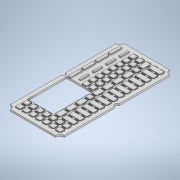
# Autodesk Inventor part: Backboard
Saved by Autodesk Inventor 2021 (Build 250183000, 183)
## iProperties
Created: 2020-06-05
Part Number: Backboard
Material: Generic
Document SubType Name: Modeling
Designer: ameli
Density: 1 g/cm^3
Appearance: Default
Author: ameli
Autodesk Inventor part; units mm, degrees
(part 1 of 3)
ref_plane "YZ Plane" through (0, 0, 0) normal (1, 0, 0) x (0, 1, 0)
ref_plane "XZ Plane" through (0, 0, 0) normal (0, 1, 0) x (-1, 0, 0)
ref_plane "XY Plane" through (0, 0, 0) normal (0, 0, 1) x (1, 0, 0)
sketch "Sketch1" plane through (0, 0, 0) normal (0, 1, 0) x (-1, 0, 0)
  line L0 (60.5, 128.5) -> (-60.5, 128.5)
  line L1 (-60.5, 128.5) -> (-60.5, -128.5)
  line L2 (-60.5, -128.5) -> (60.5, -128.5)
  line L3 (60.5, -128.5) -> (60.5, 128.5)
  point P0 (0, 0)
  dimension "d0" = 121
  dimension "d1" = 257
  dimension "d2" = 60.5
  dimension "d3" = 128.5
  constraints: 8 end point, 2 parallel, 1 horizontal, 1 perpendicular
  measures "d0" distance of L0.start L0.end
  measures "d1" distance of L2.end L0.start
  measures "d2" distance from line of point (0, 0) L3
  measures "d3" distance from line of point (0, 0) L0
extrude "Extrusion1" add sketch "Sketch1" along normal blind 4
sketch "Sketch6" plane through (0, 4, 0) normal (0, 1, 0) x (1, 0, 0)
  line L0 (-52, -89.5) -> (7, -89.5)
  line L1 (7, -89.5) -> (7, -0.5)
  line L2 (7, -0.5) -> (-52, -0.5)
  line L3 (-52, -0.5) -> (-52, -89.5)
  line L4 (-60.5, 128.5) -> (-60.5, -128.5) projected
  line L5 (-60.5, -128.5) -> (60.5, -128.5) projected
  point P0 (0, 0)
  dimension "d22" = 89
  dimension "d23" = 59
  dimension "d24" = 8.5
  dimension "d336" = 39
  constraints: 8 end point, 2 parallel, 1 horizontal, 1 perpendicular
  measures "d22" distance of L2.end L0.start
  measures "d23" distance of L0.start L0.end
  measures "d24" distance between parallel lines of L4 L3
  measures "d336" distance between parallel lines of L5 L0
extrude "Extrusion2" cut sketch "Sketch6" against normal blind 10
sketch "Sketch10" plane through (0, 4, 0) normal (0, 1, 0) x (1, 0, 0)
  line L0 (-49.25, -119.5) -> (-40.75, -119.5)
  line L1 (-40.75, -119.5) -> (-40.75, -118)
  line L2 (-40.75, -118) -> (-49.25, -118)
  line L3 (-49.25, -118) -> (-49.25, -119.5)
  line L4 (-49.25, -107) -> (-40.75, -107)
  line L5 (-40.75, -107) -> (-40.75, -105.5)
  line L6 (-40.75, -105.5) -> (-49.25, -105.5)
  line L7 (-49.25, -105.5) -> (-49.25, -107)
  line L8 (-60.5, 128.5) -> (-60.5, -128.5) projected
  line L9 (-60.5, -128.5) -> (60.5, -128.5) projected
  line L10 (-49.25, -104.5) -> (-40.75, -104.5)
  line L11 (-40.75, -104.5) -> (-40.75, -103)
  line L12 (-40.75, -103) -> (-49.25, -103)
  line L13 (-49.25, -103) -> (-49.25, -104.5)
  line L14 (-49.25, -92) -> (-40.75, -92)
  line L15 (-40.75, -92) -> (-40.75, -90.5)
  line L16 (-40.75, -90.5) -> (-49.25, -90.5)
  line L17 (-49.25, -90.5) -> (-49.25, -92)
  line L18 (-49.25, -89.5) -> (-40.75, -89.5)
  line L19 (-40.75, -89.5) -> (-40.75, -88)
  line L20 (-40.75, -88) -> (-49.25, -88)
  line L21 (-49.25, -88) -> (-49.25, -89.5)
  line L22 (-49.25, -77) -> (-40.75, -77)
  line L23 (-40.75, -77) -> (-40.75, -75.5)
  line L24 (-40.75, -75.5) -> (-49.25, -75.5)
  line L25 (-49.25, -75.5) -> (-49.25, -77)
  line L26 (-49.25, -74.5) -> (-40.75, -74.5)
  line L27 (-40.75, -74.5) -> (-40.75, -73)
  line L28 (-40.75, -73) -> (-49.25, -73)
  line L29 (-49.25, -73) -> (-49.25, -74.5)
  line L30 (-49.25, -62) -> (-40.75, -62)
  line L31 (-40.75, -62) -> (-40.75, -60.5)
  line L32 (-40.75, -60.5) -> (-49.25, -60.5)
  line L33 (-49.25, -60.5) -> (-49.25, -62)
  line L34 (-49.25, -59.5) -> (-40.75, -59.5)
  line L35 (-40.75, -59.5) -> (-40.75, -58)
  line L36 (-40.75, -58) -> (-49.25, -58)
  line L37 (-49.25, -58) -> (-49.25, -59.5)
  line L38 (-49.25, -47) -> (-40.75, -47)
  line L39 (-40.75, -47) -> (-40.75, -45.5)
  line L40 (-40.75, -45.5) -> (-49.25, -45.5)
  line L41 (-49.25, -45.5) -> (-49.25, -47)
  line L42 (-49.25, -44.5) -> (-40.75, -44.5)
  line L43 (-40.75, -44.5) -> (-40.75, -43)
  line L44 (-40.75, -43) -> (-49.25, -43)
  line L45 (-49.25, -43) -> (-49.25, -44.5)
  line L46 (-49.25, -32) -> (-40.75, -32)
  line L47 (-40.75, -32) -> (-40.75, -30.5)
  line L48 (-40.75, -30.5) -> (-49.25, -30.5)
  line L49 (-49.25, -30.5) -> (-49.25, -32)
  line L50 (-49.25, -29.5) -> (-40.75, -29.5)
  line L51 (-40.75, -29.5) -> (-40.75, -28)
  line L52 (-40.75, -28) -> (-49.25, -28)
  line L53 (-49.25, -28) -> (-49.25, -29.5)
  line L54 (-49.25, -17) -> (-40.75, -17)
  line L55 (-40.75, -17) -> (-40.75, -15.5)
  line L56 (-40.75, -15.5) -> (-49.25, -15.5)
  line L57 (-49.25, -15.5) -> (-49.25, -17)
  line L58 (-49.25, -14.5) -> (-40.75, -14.5)
  line L59 (-40.75, -14.5) -> (-40.75, -13)
  line L60 (-40.75, -13) -> (-49.25, -13)
  line L61 (-49.25, -13) -> (-49.25, -14.5)
  line L62 (-49.25, -2) -> (-40.75, -2)
  line L63 (-40.75, -2) -> (-40.75, -0.5)
  line L64 (-40.75, -0.5) -> (-49.25, -0.5)
  line L65 (-49.25, -0.5) -> (-49.25, -2)
  line L66 (-49.25, 0.5) -> (-40.75, 0.5)
  line L67 (-40.75, 0.5) -> (-40.75, 2)
  line L68 (-40.75, 2) -> (-49.25, 2)
  line L69 (-49.25, 2) -> (-49.25, 0.5)
  line L70 (-49.25, 13) -> (-40.75, 13)
  line L71 (-40.75, 13) -> (-40.75, 14.5)
  line L72 (-40.75, 14.5) -> (-49.25, 14.5)
  line L73 (-49.25, 14.5) -> (-49.25, 13)
  line L74 (-49.25, 15.5) -> (-40.75, 15.5)
  line L75 (-40.75, 15.5) -> (-40.75, 17)
  line L76 (-40.75, 17) -> (-49.25, 17)
  line L77 (-49.25, 17) -> (-49.25, 15.5)
  line L78 (-49.25, 28) -> (-40.75, 28)
  line L79 (-40.75, 28) -> (-40.75, 29.5)
  line L80 (-40.75, 29.5) -> (-49.25, 29.5)
  line L81 (-49.25, 29.5) -> (-49.25, 28)
  line L82 (-49.25, 30.5) -> (-40.75, 30.5)
  line L83 (-40.75, 30.5) -> (-40.75, 32)
  line L84 (-40.75, 32) -> (-49.25, 32)
  line L85 (-49.25, 32) -> (-49.25, 30.5)
  line L86 (-49.25, 43) -> (-40.75, 43)
  line L87 (-40.75, 43) -> (-40.75, 44.5)
  line L88 (-40.75, 44.5) -> (-49.25, 44.5)
  line L89 (-49.25, 44.5) -> (-49.25, 43)
  line L90 (-49.25, 45.5) -> (-40.75, 45.5)
  line L91 (-40.75, 45.5) -> (-40.75, 47)
  line L92 (-40.75, 47) -> (-49.25, 47)
  line L93 (-49.25, 47) -> (-49.25, 45.5)
  line L94 (-49.25, 58) -> (-40.75, 58)
  line L95 (-40.75, 58) -> (-40.75, 59.5)
  line L96 (-40.75, 59.5) -> (-49.25, 59.5)
  line L97 (-49.25, 59.5) -> (-49.25, 58)
  line L98 (-49.25, 60.5) -> (-40.75, 60.5)
  line L99 (-40.75, 60.5) -> (-40.75, 62)
  line L100 (-40.75, 62) -> (-49.25, 62)
  line L101 (-49.25, 62) -> (-49.25, 60.5)
  line L102 (-49.25, 73) -> (-40.75, 73)
  line L103 (-40.75, 73) -> (-40.75, 74.5)
  line L104 (-40.75, 74.5) -> (-49.25, 74.5)
  line L105 (-49.25, 74.5) -> (-49.25, 73)
  line L106 (-49.25, 75.5) -> (-40.75, 75.5)
  line L107 (-40.75, 75.5) -> (-40.75, 77)
  line L108 (-40.75, 77) -> (-49.25, 77)
  line L109 (-49.25, 77) -> (-49.25, 75.5)
  line L110 (-49.25, 88) -> (-40.75, 88)
  line L111 (-40.75, 88) -> (-40.75, 89.5)
  line L112 (-40.75, 89.5) -> (-49.25, 89.5)
  line L113 (-49.25, 89.5) -> (-49.25, 88)
  line L114 (-49.25, 90.5) -> (-40.75, 90.5)
  line L115 (-40.75, 90.5) -> (-40.75, 92)
  line L116 (-40.75, 92) -> (-49.25, 92)
  line L117 (-49.25, 92) -> (-49.25, 90.5)
  line L118 (-49.25, 103) -> (-40.75, 103)
  line L119 (-40.75, 103) -> (-40.75, 104.5)
  line L120 (-40.75, 104.5) -> (-49.25, 104.5)
  line L121 (-49.25, 104.5) -> (-49.25, 103)
  line L122 (-49.25, 105.5) -> (-40.75, 105.5)
  line L123 (-40.75, 105.5) -> (-40.75, 107)
  line L124 (-40.75, 107) -> (-49.25, 107)
  line L125 (-49.25, 107) -> (-49.25, 105.5)
  line L126 (-49.25, 118) -> (-40.75, 118)
  line L127 (-40.75, 118) -> (-40.75, 119.5)
  line L128 (-40.75, 119.5) -> (-49.25, 119.5)
  line L129 (-49.25, 119.5) -> (-49.25, 118)
  line L130 (-34.25, -119.5) -> (-25.75, -119.5)
  line L131 (-25.75, -119.5) -> (-25.75, -118)
  line L132 (-25.75, -118) -> (-34.25, -118)
  line L133 (-34.25, -118) -> (-34.25, -119.5)
  line L134 (-34.25, -107) -> (-25.75, -107)
  line L135 (-25.75, -107) -> (-25.75, -105.5)
  line L136 (-25.75, -105.5) -> (-34.25, -105.5)
  line L137 (-34.25, -105.5) -> (-34.25, -107)
  line L138 (-34.25, -104.5) -> (-25.75, -104.5)
  line L139 (-25.75, -104.5) -> (-25.75, -103)
  line L140 (-25.75, -103) -> (-34.25, -103)
  line L141 (-34.25, -103) -> (-34.25, -104.5)
  line L142 (-34.25, -92) -> (-25.75, -92)
  line L143 (-25.75, -92) -> (-25.75, -90.5)
  line L144 (-25.75, -90.5) -> (-34.25, -90.5)
  line L145 (-34.25, -90.5) -> (-34.25, -92)
  line L146 (-34.25, -89.5) -> (-25.75, -89.5)
  line L147 (-25.75, -89.5) -> (-25.75, -88)
  line L148 (-25.75, -88) -> (-34.25, -88)
  line L149 (-34.25, -88) -> (-34.25, -89.5)
  line L150 (-34.25, -77) -> (-25.75, -77)
  line L151 (-25.75, -77) -> (-25.75, -75.5)
  line L152 (-25.75, -75.5) -> (-34.25, -75.5)
  line L153 (-34.25, -75.5) -> (-34.25, -77)
  line L154 (-34.25, -74.5) -> (-25.75, -74.5)
  line L155 (-25.75, -74.5) -> (-25.75, -73)
  line L156 (-25.75, -73) -> (-34.25, -73)
  line L157 (-34.25, -73) -> (-34.25, -74.5)
  line L158 (-34.25, -62) -> (-25.75, -62)
  line L159 (-25.75, -62) -> (-25.75, -60.5)
  line L160 (-25.75, -60.5) -> (-34.25, -60.5)
  line L161 (-34.25, -60.5) -> (-34.25, -62)
  line L162 (-34.25, -59.5) -> (-25.75, -59.5)
  line L163 (-25.75, -59.5) -> (-25.75, -58)
  line L164 (-25.75, -58) -> (-34.25, -58)
  line L165 (-34.25, -58) -> (-34.25, -59.5)
  line L166 (-34.25, -47) -> (-25.75, -47)
  line L167 (-25.75, -47) -> (-25.75, -45.5)
  line L168 (-25.75, -45.5) -> (-34.25, -45.5)
  line L169 (-34.25, -45.5) -> (-34.25, -47)
  line L170 (-34.25, -44.5) -> (-25.75, -44.5)
  line L171 (-25.75, -44.5) -> (-25.75, -43)
  line L172 (-25.75, -43) -> (-34.25, -43)
  line L173 (-34.25, -43) -> (-34.25, -44.5)
  line L174 (-34.25, -32) -> (-25.75, -32)
  line L175 (-25.75, -32) -> (-25.75, -30.5)
  line L176 (-25.75, -30.5) -> (-34.25, -30.5)
  line L177 (-34.25, -30.5) -> (-34.25, -32)
  line L178 (-34.25, -29.5) -> (-25.75, -29.5)
  line L179 (-25.75, -29.5) -> (-25.75, -28)
  line L180 (-25.75, -28) -> (-34.25, -28)
  line L181 (-34.25, -28) -> (-34.25, -29.5)
  line L182 (-34.25, -17) -> (-25.75, -17)
  line L183 (-25.75, -17) -> (-25.75, -15.5)
  line L184 (-25.75, -15.5) -> (-34.25, -15.5)
  line L185 (-34.25, -15.5) -> (-34.25, -17)
  line L186 (-34.25, -14.5) -> (-25.75, -14.5)
  line L187 (-25.75, -14.5) -> (-25.75, -13)
  line L188 (-25.75, -13) -> (-34.25, -13)
  line L189 (-34.25, -13) -> (-34.25, -14.5)
  line L190 (-34.25, -2) -> (-25.75, -2)
  line L191 (-25.75, -2) -> (-25.75, -0.5)
  line L192 (-25.75, -0.5) -> (-34.25, -0.5)
  line L193 (-34.25, -0.5) -> (-34.25, -2)
  line L194 (-34.25, 0.5) -> (-25.75, 0.5)
  line L195 (-25.75, 0.5) -> (-25.75, 2)
  line L196 (-25.75, 2) -> (-34.25, 2)
  line L197 (-34.25, 2) -> (-34.25, 0.5)
  line L198 (-34.25, 13) -> (-25.75, 13)
  line L199 (-25.75, 13) -> (-25.75, 14.5)
  line L200 (-25.75, 14.5) -> (-34.25, 14.5)
  line L201 (-34.25, 14.5) -> (-34.25, 13)
  line L202 (-34.25, 15.5) -> (-25.75, 15.5)
  line L203 (-25.75, 15.5) -> (-25.75, 17)
  line L204 (-25.75, 17) -> (-34.25, 17)
  line L205 (-34.25, 17) -> (-34.25, 15.5)
  line L206 (-34.25, 28) -> (-25.75, 28)
  line L207 (-25.75, 28) -> (-25.75, 29.5)
  line L208 (-25.75, 29.5) -> (-34.25, 29.5)
  line L209 (-34.25, 29.5) -> (-34.25, 28)
  line L210 (-34.25, 30.5) -> (-25.75, 30.5)
  line L211 (-25.75, 30.5) -> (-25.75, 32)
  line L212 (-25.75, 32) -> (-34.25, 32)
  line L213 (-34.25, 32) -> (-34.25, 30.5)
  line L214 (-34.25, 43) -> (-25.75, 43)
  line L215 (-25.75, 43) -> (-25.75, 44.5)
  line L216 (-25.75, 44.5) -> (-34.25, 44.5)
  line L217 (-34.25, 44.5) -> (-34.25, 43)
  line L218 (-34.25, 45.5) -> (-25.75, 45.5)
  line L219 (-25.75, 45.5) -> (-25.75, 47)
  line L220 (-25.75, 47) -> (-34.25, 47)
  line L221 (-34.25, 47) -> (-34.25, 45.5)
  line L222 (-34.25, 58) -> (-25.75, 58)
  line L223 (-25.75, 58) -> (-25.75, 59.5)
  line L224 (-25.75, 59.5) -> (-34.25, 59.5)
  line L225 (-34.25, 59.5) -> (-34.25, 58)
  line L226 (-34.25, 60.5) -> (-25.75, 60.5)
  line L227 (-25.75, 60.5) -> (-25.75, 62)
  line L228 (-25.75, 62) -> (-34.25, 62)
  line L229 (-34.25, 62) -> (-34.25, 60.5)
  line L230 (-34.25, 73) -> (-25.75, 73)
  line L231 (-25.75, 73) -> (-25.75, 74.5)
  line L232 (-25.75, 74.5) -> (-34.25, 74.5)
  line L233 (-34.25, 74.5) -> (-34.25, 73)
  line L234 (-34.25, 75.5) -> (-25.75, 75.5)
  line L235 (-25.75, 75.5) -> (-25.75, 77)
  line L236 (-25.75, 77) -> (-34.25, 77)
  line L237 (-34.25, 77) -> (-34.25, 75.5)
  line L238 (-34.25, 88) -> (-25.75, 88)
  line L239 (-25.75, 88) -> (-25.75, 89.5)
  line L240 (-25.75, 89.5) -> (-34.25, 89.5)
  line L241 (-34.25, 89.5) -> (-34.25, 88)
  line L242 (-34.25, 90.5) -> (-25.75, 90.5)
  line L243 (-25.75, 90.5) -> (-25.75, 92)
  line L244 (-25.75, 92) -> (-34.25, 92)
  line L245 (-34.25, 92) -> (-34.25, 90.5)
  line L246 (-34.25, 103) -> (-25.75, 103)
  line L247 (-25.75, 103) -> (-25.75, 104.5)
  line L248 (-25.75, 104.5) -> (-34.25, 104.5)
  line L249 (-34.25, 104.5) -> (-34.25, 103)
  line L250 (-34.25, 105.5) -> (-25.75, 105.5)
  line L251 (-25.75, 105.5) -> (-25.75, 107)
  line L252 (-25.75, 107) -> (-34.25, 107)
  line L253 (-34.25, 107) -> (-34.25, 105.5)
  line L254 (-34.25, 118) -> (-25.75, 118)
  line L255 (-25.75, 118) -> (-25.75, 119.5)
  line L256 (-25.75, 119.5) -> (-34.25, 119.5)
  line L257 (-34.25, 119.5) -> (-34.25, 118)
  line L258 (-19.25, -119.5) -> (-10.75, -119.5)
  line L259 (-10.75, -119.5) -> (-10.75, -118)
  line L260 (-10.75, -118) -> (-19.25, -118)
  line L261 (-19.25, -118) -> (-19.25, -119.5)
  line L262 (-19.25, -107) -> (-10.75, -107)
  line L263 (-10.75, -107) -> (-10.75, -105.5)
  line L264 (-10.75, -105.5) -> (-19.25, -105.5)
  line L265 (-19.25, -105.5) -> (-19.25, -107)
  line L266 (-19.25, -104.5) -> (-10.75, -104.5)
  line L267 (-10.75, -104.5) -> (-10.75, -103)
  line L268 (-10.75, -103) -> (-19.25, -103)
  line L269 (-19.25, -103) -> (-19.25, -104.5)
  line L270 (-19.25, -92) -> (-10.75, -92)
  line L271 (-10.75, -92) -> (-10.75, -90.5)
  line L272 (-10.75, -90.5) -> (-19.25, -90.5)
  line L273 (-19.25, -90.5) -> (-19.25, -92)
  line L274 (-19.25, -89.5) -> (-10.75, -89.5)
  line L275 (-10.75, -89.5) -> (-10.75, -88)
  line L276 (-10.75, -88) -> (-19.25, -88)
  line L277 (-19.25, -88) -> (-19.25, -89.5)
  line L278 (-19.25, -77) -> (-10.75, -77)
  line L279 (-10.75, -77) -> (-10.75, -75.5)
  line L280 (-10.75, -75.5) -> (-19.25, -75.5)
  line L281 (-19.25, -75.5) -> (-19.25, -77)
  line L282 (-19.25, -74.5) -> (-10.75, -74.5)
  line L283 (-10.75, -74.5) -> (-10.75, -73)
  line L284 (-10.75, -73) -> (-19.25, -73)
  line L285 (-19.25, -73) -> (-19.25, -74.5)
  line L286 (-19.25, -62) -> (-10.75, -62)
  line L287 (-10.75, -62) -> (-10.75, -60.5)
  line L288 (-10.75, -60.5) -> (-19.25, -60.5)
  line L289 (-19.25, -60.5) -> (-19.25, -62)
  line L290 (-19.25, -59.5) -> (-10.75, -59.5)
  line L291 (-10.75, -59.5) -> (-10.75, -58)
  line L292 (-10.75, -58) -> (-19.25, -58)
  line L293 (-19.25, -58) -> (-19.25, -59.5)
  line L294 (-19.25, -47) -> (-10.75, -47)
  line L295 (-10.75, -47) -> (-10.75, -45.5)
  line L296 (-10.75, -45.5) -> (-19.25, -45.5)
  line L297 (-19.25, -45.5) -> (-19.25, -47)
  line L298 (-19.25, -44.5) -> (-10.75, -44.5)
  line L299 (-10.75, -44.5) -> (-10.75, -43)
  line L300 (-10.75, -43) -> (-19.25, -43)
  line L301 (-19.25, -43) -> (-19.25, -44.5)
  line L302 (-19.25, -32) -> (-10.75, -32)
  line L303 (-10.75, -32) -> (-10.75, -30.5)
  line L304 (-10.75, -30.5) -> (-19.25, -30.5)
  line L305 (-19.25, -30.5) -> (-19.25, -32)
  line L306 (-19.25, -29.5) -> (-10.75, -29.5)
  line L307 (-10.75, -29.5) -> (-10.75, -28)
  line L308 (-10.75, -28) -> (-19.25, -28)
  line L309 (-19.25, -28) -> (-19.25, -29.5)
  line L310 (-19.25, -17) -> (-10.75, -17)
  line L311 (-10.75, -17) -> (-10.75, -15.5)
  line L312 (-10.75, -15.5) -> (-19.25, -15.5)
  line L313 (-19.25, -15.5) -> (-19.25, -17)
  line L314 (-19.25, -14.5) -> (-10.75, -14.5)
  line L315 (-10.75, -14.5) -> (-10.75, -13)
  line L316 (-10.75, -13) -> (-19.25, -13)
  line L317 (-19.25, -13) -> (-19.25, -14.5)
  line L318 (-19.25, -2) -> (-10.75, -2)
  line L319 (-10.75, -2) -> (-10.75, -0.5)
  line L320 (-10.75, -0.5) -> (-19.25, -0.5)
  line L321 (-19.25, -0.5) -> (-19.25, -2)
  line L322 (-19.25, 0.5) -> (-10.75, 0.5)
  line L323 (-10.75, 0.5) -> (-10.75, 2)
  line L324 (-10.75, 2) -> (-19.25, 2)
  line L325 (-19.25, 2) -> (-19.25, 0.5)
  line L326 (-19.25, 13) -> (-10.75, 13)
  line L327 (-10.75, 13) -> (-10.75, 14.5)
  line L328 (-10.75, 14.5) -> (-19.25, 14.5)
  line L329 (-19.25, 14.5) -> (-19.25, 13)
  line L330 (-19.25, 15.5) -> (-10.75, 15.5)
  line L331 (-10.75, 15.5) -> (-10.75, 17)
  line L332 (-10.75, 17) -> (-19.25, 17)
  line L333 (-19.25, 17) -> (-19.25, 15.5)
  line L334 (-19.25, 28) -> (-10.75, 28)
  line L335 (-10.75, 28) -> (-10.75, 29.5)
  line L336 (-10.75, 29.5) -> (-19.25, 29.5)
  line L337 (-19.25, 29.5) -> (-19.25, 28)
  line L338 (-19.25, 30.5) -> (-10.75, 30.5)
  line L339 (-10.75, 30.5) -> (-10.75, 32)
  line L340 (-10.75, 32) -> (-19.25, 32)
  line L341 (-19.25, 32) -> (-19.25, 30.5)
  line L342 (-19.25, 43) -> (-10.75, 43)
  line L343 (-10.75, 43) -> (-10.75, 44.5)
  line L344 (-10.75, 44.5) -> (-19.25, 44.5)
  line L345 (-19.25, 44.5) -> (-19.25, 43)
  line L346 (-19.25, 45.5) -> (-10.75, 45.5)
  line L347 (-10.75, 45.5) -> (-10.75, 47)
  line L348 (-10.75, 47) -> (-19.25, 47)
  line L349 (-19.25, 47) -> (-19.25, 45.5)
  line L350 (-19.25, 58) -> (-10.75, 58)
  line L351 (-10.75, 58) -> (-10.75, 59.5)
  line L352 (-10.75, 59.5) -> (-19.25, 59.5)
  line L353 (-19.25, 59.5) -> (-19.25, 58)
  line L354 (-19.25, 60.5) -> (-10.75, 60.5)
  line L355 (-10.75, 60.5) -> (-10.75, 62)
  line L356 (-10.75, 62) -> (-19.25, 62)
  line L357 (-19.25, 62) -> (-19.25, 60.5)
  line L358 (-19.25, 73) -> (-10.75, 73)
  line L359 (-10.75, 73) -> (-10.75, 74.5)
  line L360 (-10.75, 74.5) -> (-19.25, 74.5)
  line L361 (-19.25, 74.5) -> (-19.25, 73)
  line L362 (-19.25, 75.5) -> (-10.75, 75.5)
  line L363 (-10.75, 75.5) -> (-10.75, 77)
  line L364 (-10.75, 77) -> (-19.25, 77)
  line L365 (-19.25, 77) -> (-19.25, 75.5)
  line L366 (-19.25, 88) -> (-10.75, 88)
  line L367 (-10.75, 88) -> (-10.75, 89.5)
  line L368 (-10.75, 89.5) -> (-19.25, 89.5)
  line L369 (-19.25, 89.5) -> (-19.25, 88)
  line L370 (-19.25, 90.5) -> (-10.75, 90.5)
  line L371 (-10.75, 90.5) -> (-10.75, 92)
  line L372 (-10.75, 92) -> (-19.25, 92)
  line L373 (-19.25, 92) -> (-19.25, 90.5)
  line L374 (-19.25, 103) -> (-10.75, 103)
  line L375 (-10.75, 103) -> (-10.75, 104.5)
  line L376 (-10.75, 104.5) -> (-19.25, 104.5)
  line L377 (-19.25, 104.5) -> (-19.25, 103)
  line L378 (-19.25, 105.5) -> (-10.75, 105.5)
  line L379 (-10.75, 105.5) -> (-10.75, 107)
  line L380 (-10.75, 107) -> (-19.25, 107)
  line L381 (-19.25, 107) -> (-19.25, 105.5)
  line L382 (-19.25, 118) -> (-10.75, 118)
  line L383 (-10.75, 118) -> (-10.75, 119.5)
  line L384 (-10.75, 119.5) -> (-19.25, 119.5)
  line L385 (-19.25, 119.5) -> (-19.25, 118)
  line L386 (-4.25, -119.5) -> (4.25, -119.5)
  line L387 (4.25, -119.5) -> (4.25, -118)
  line L388 (4.25, -118) -> (-4.25, -118)
  line L389 (-4.25, -118) -> (-4.25, -119.5)
  line L390 (-4.25, -107) -> (4.25, -107)
  line L391 (4.25, -107) -> (4.25, -105.5)
  line L392 (4.25, -105.5) -> (-4.25, -105.5)
  line L393 (-4.25, -105.5) -> (-4.25, -107)
  line L394 (-4.25, -104.5) -> (4.25, -104.5)
  line L395 (4.25, -104.5) -> (4.25, -103)
  line L396 (4.25, -103) -> (-4.25, -103)
  line L397 (-4.25, -103) -> (-4.25, -104.5)
  line L398 (-4.25, -92) -> (4.25, -92)
  line L399 (4.25, -92) -> (4.25, -90.5)
  line L400 (4.25, -90.5) -> (-4.25, -90.5)
  line L401 (-4.25, -90.5) -> (-4.25, -92)
  line L402 (-4.25, -89.5) -> (4.25, -89.5)
  line L403 (4.25, -89.5) -> (4.25, -88)
  line L404 (4.25, -88) -> (-4.25, -88)
  line L405 (-4.25, -88) -> (-4.25, -89.5)
  line L406 (-4.25, -77) -> (4.25, -77)
  line L407 (4.25, -77) -> (4.25, -75.5)
  line L408 (4.25, -75.5) -> (-4.25, -75.5)
  line L409 (-4.25, -75.5) -> (-4.25, -77)
  line L410 (-4.25, -74.5) -> (4.25, -74.5)
  line L411 (4.25, -74.5) -> (4.25, -73)
  line L412 (4.25, -73) -> (-4.25, -73)
  line L413 (-4.25, -73) -> (-4.25, -74.5)
  line L414 (-4.25, -62) -> (4.25, -62)
  line L415 (4.25, -62) -> (4.25, -60.5)
  line L416 (4.25, -60.5) -> (-4.25, -60.5)
  line L417 (-4.25, -60.5) -> (-4.25, -62)
  line L418 (-4.25, -59.5) -> (4.25, -59.5)
  line L419 (4.25, -59.5) -> (4.25, -58)
  line L420 (4.25, -58) -> (-4.25, -58)
  line L421 (-4.25, -58) -> (-4.25, -59.5)
  line L422 (-4.25, -47) -> (4.25, -47)
  line L423 (4.25, -47) -> (4.25, -45.5)
  line L424 (4.25, -45.5) -> (-4.25, -45.5)
  line L425 (-4.25, -45.5) -> (-4.25, -47)
  line L426 (-4.25, -44.5) -> (4.25, -44.5)
  line L427 (4.25, -44.5) -> (4.25, -43)
  line L428 (4.25, -43) -> (-4.25, -43)
  line L429 (-4.25, -43) -> (-4.25, -44.5)
  line L430 (-4.25, -32) -> (4.25, -32)
  line L431 (4.25, -32) -> (4.25, -30.5)
  line L432 (4.25, -30.5) -> (-4.25, -30.5)
  line L433 (-4.25, -30.5) -> (-4.25, -32)
  line L434 (-4.25, -29.5) -> (4.25, -29.5)
  line L435 (4.25, -29.5) -> (4.25, -28)
  line L436 (4.25, -28) -> (-4.25, -28)
  line L437 (-4.25, -28) -> (-4.25, -29.5)
  line L438 (-4.25, -17) -> (4.25, -17)
  line L439 (4.25, -17) -> (4.25, -15.5)
  line L440 (4.25, -15.5) -> (-4.25, -15.5)
  line L441 (-4.25, -15.5) -> (-4.25, -17)
  line L442 (-4.25, -14.5) -> (4.25, -14.5)
  line L443 (4.25, -14.5) -> (4.25, -13)
  line L444 (4.25, -13) -> (-4.25, -13)
  line L445 (-4.25, -13) -> (-4.25, -14.5)
  line L446 (-4.25, -2) -> (4.25, -2)
  line L447 (4.25, -2) -> (4.25, -0.5)
  line L448 (4.25, -0.5) -> (-4.25, -0.5)
  line L449 (-4.25, -0.5) -> (-4.25, -2)
  line L450 (-4.25, 0.5) -> (4.25, 0.5)
  line L451 (4.25, 0.5) -> (4.25, 2)
  line L452 (4.25, 2) -> (-4.25, 2)
  line L453 (-4.25, 2) -> (-4.25, 0.5)
  line L454 (-4.25, 13) -> (4.25, 13)
  line L455 (4.25, 13) -> (4.25, 14.5)
  line L456 (4.25, 14.5) -> (-4.25, 14.5)
  line L457 (-4.25, 14.5) -> (-4.25, 13)
  line L458 (-4.25, 15.5) -> (4.25, 15.5)
  line L459 (4.25, 15.5) -> (4.25, 17)
  line L460 (4.25, 17) -> (-4.25, 17)
  line L461 (-4.25, 17) -> (-4.25, 15.5)
  line L462 (-4.25, 28) -> (4.25, 28)
  line L463 (4.25, 28) -> (4.25, 29.5)
  line L464 (4.25, 29.5) -> (-4.25, 29.5)
  line L465 (-4.25, 29.5) -> (-4.25, 28)
  line L466 (-4.25, 30.5) -> (4.25, 30.5)
  line L467 (4.25, 30.5) -> (4.25, 32)
  line L468 (4.25, 32) -> (-4.25, 32)
  line L469 (-4.25, 32) -> (-4.25, 30.5)
  line L470 (-4.25, 43) -> (4.25, 43)
  line L471 (4.25, 43) -> (4.25, 44.5)
  line L472 (4.25, 44.5) -> (-4.25, 44.5)
  line L473 (-4.25, 44.5) -> (-4.25, 43)
  line L474 (-4.25, 45.5) -> (4.25, 45.5)
  line L475 (4.25, 45.5) -> (4.25, 47)
  line L476 (4.25, 47) -> (-4.25, 47)
  line L477 (-4.25, 47) -> (-4.25, 45.5)
  line L478 (-4.25, 58) -> (4.25, 58)
  line L479 (4.25, 58) -> (4.25, 59.5)
  line L480 (4.25, 59.5) -> (-4.25, 59.5)
  line L481 (-4.25, 59.5) -> (-4.25, 58)
  line L482 (-4.25, 60.5) -> (4.25, 60.5)
  line L483 (4.25, 60.5) -> (4.25, 62)
  line L484 (4.25, 62) -> (-4.25, 62)
  line L485 (-4.25, 62) -> (-4.25, 60.5)
  line L486 (-4.25, 73) -> (4.25, 73)
  line L487 (4.25, 73) -> (4.25, 74.5)
  line L488 (4.25, 74.5) -> (-4.25, 74.5)
  line L489 (-4.25, 74.5) -> (-4.25, 73)
  line L490 (-4.25, 75.5) -> (4.25, 75.5)
  line L491 (4.25, 75.5) -> (4.25, 77)
  line L492 (4.25, 77) -> (-4.25, 77)
  line L493 (-4.25, 77) -> (-4.25, 75.5)
  line L494 (-4.25, 88) -> (4.25, 88)
  line L495 (4.25, 88) -> (4.25, 89.5)
  line L496 (4.25, 89.5) -> (-4.25, 89.5)
  line L497 (-4.25, 89.5) -> (-4.25, 88)
  line L498 (-4.25, 90.5) -> (4.25, 90.5)
  line L499 (4.25, 90.5) -> (4.25, 92)
  line L500 (4.25, 92) -> (-4.25, 92)
  line L501 (-4.25, 92) -> (-4.25, 90.5)
  line L502 (-4.25, 103) -> (4.25, 103)
  line L503 (4.25, 103) -> (4.25, 104.5)
  line L504 (4.25, 104.5) -> (-4.25, 104.5)
  line L505 (-4.25, 104.5) -> (-4.25, 103)
  line L506 (-4.25, 105.5) -> (4.25, 105.5)
  line L507 (4.25, 105.5) -> (4.25, 107)
  line L508 (4.25, 107) -> (-4.25, 107)
  line L509 (-4.25, 107) -> (-4.25, 105.5)
  line L510 (-4.25, 118) -> (4.25, 118)
  line L511 (4.25, 118) -> (4.25, 119.5)
  line L512 (4.25, 119.5) -> (-4.25, 119.5)
  line L513 (-4.25, 119.5) -> (-4.25, 118)
  line L514 (10.75, -119.5) -> (19.25, -119.5)
  line L515 (19.25, -119.5) -> (19.25, -118)
  line L516 (19.25, -118) -> (10.75, -118)
  line L517 (10.75, -118) -> (10.75, -119.5)
  line L518 (10.75, -107) -> (19.25, -107)
  line L519 (19.25, -107) -> (19.25, -105.5)
  line L520 (19.25, -105.5) -> (10.75, -105.5)
  line L521 (10.75, -105.5) -> (10.75, -107)
  line L522 (10.75, -104.5) -> (19.25, -104.5)
  line L523 (19.25, -104.5) -> (19.25, -103)
  line L524 (19.25, -103) -> (10.75, -103)
  line L525 (10.75, -103) -> (10.75, -104.5)
  line L526 (10.75, -92) -> (19.25, -92)
  line L527 (19.25, -92) -> (19.25, -90.5)
  line L528 (19.25, -90.5) -> (10.75, -90.5)
  line L529 (10.75, -90.5) -> (10.75, -92)
  line L530 (10.75, -89.5) -> (19.25, -89.5)
  line L531 (19.25, -89.5) -> (19.25, -88)
  line L532 (19.25, -88) -> (10.75, -88)
  line L533 (10.75, -88) -> (10.75, -89.5)
  line L534 (10.75, -77) -> (19.25, -77)
  line L535 (19.25, -77) -> (19.25, -75.5)
  line L536 (19.25, -75.5) -> (10.75, -75.5)
  line L537 (10.75, -75.5) -> (10.75, -77)
  line L538 (10.75, -74.5) -> (19.25, -74.5)
  line L539 (19.25, -74.5) -> (19.25, -73)
  line L540 (19.25, -73) -> (10.75, -73)
  line L541 (10.75, -73) -> (10.75, -74.5)
  line L542 (10.75, -62) -> (19.25, -62)
  line L543 (19.25, -62) -> (19.25, -60.5)
  line L544 (19.25, -60.5) -> (10.75, -60.5)
  line L545 (10.75, -60.5) -> (10.75, -62)
  line L546 (10.75, -59.5) -> (19.25, -59.5)
  line L547 (19.25, -59.5) -> (19.25, -58)
  line L548 (19.25, -58) -> (10.75, -58)
  line L549 (10.75, -58) -> (10.75, -59.5)
  line L550 (10.75, -47) -> (19.25, -47)
  line L551 (19.25, -47) -> (19.25, -45.5)
  line L552 (19.25, -45.5) -> (10.75, -45.5)
  line L553 (10.75, -45.5) -> (10.75, -47)
  line L554 (10.75, -44.5) -> (19.25, -44.5)
  line L555 (19.25, -44.5) -> (19.25, -43)
  line L556 (19.25, -43) -> (10.75, -43)
  line L557 (10.75, -43) -> (10.75, -44.5)
  line L558 (10.75, -32) -> (19.25, -32)
  line L559 (19.25, -32) -> (19.25, -30.5)
  line L560 (19.25, -30.5) -> (10.75, -30.5)
  line L561 (10.75, -30.5) -> (10.75, -32)
  line L562 (10.75, -29.5) -> (19.25, -29.5)
  line L563 (19.25, -29.5) -> (19.25, -28)
  line L564 (19.25, -28) -> (10.75, -28)
  line L565 (10.75, -28) -> (10.75, -29.5)
  line L566 (10.75, -17) -> (19.25, -17)
  line L567 (19.25, -17) -> (19.25, -15.5)
  line L568 (19.25, -15.5) -> (10.75, -15.5)
  line L569 (10.75, -15.5) -> (10.75, -17)
  line L570 (10.75, -14.5) -> (19.25, -14.5)
  line L571 (19.25, -14.5) -> (19.25, -13)
  line L572 (19.25, -13) -> (10.75, -13)
  line L573 (10.75, -13) -> (10.75, -14.5)
  line L574 (10.75, -2) -> (19.25, -2)
  line L575 (19.25, -2) -> (19.25, -0.5)
  line L576 (19.25, -0.5) -> (10.75, -0.5)
  line L577 (10.75, -0.5) -> (10.75, -2)
  line L578 (10.75, 0.5) -> (19.25, 0.5)
  line L579 (19.25, 0.5) -> (19.25, 2)
  line L580 (19.25, 2) -> (10.75, 2)
  line L581 (10.75, 2) -> (10.75, 0.5)
  line L582 (10.75, 13) -> (19.25, 13)
  line L583 (19.25, 13) -> (19.25, 14.5)
  line L584 (19.25, 14.5) -> (10.75, 14.5)
  line L585 (10.75, 14.5) -> (10.75, 13)
  line L586 (10.75, 15.5) -> (19.25, 15.5)
  line L587 (19.25, 15.5) -> (19.25, 17)
  line L588 (19.25, 17) -> (10.75, 17)
  line L589 (10.75, 17) -> (10.75, 15.5)
  line L590 (10.75, 28) -> (19.25, 28)
  line L591 (19.25, 28) -> (19.25, 29.5)
  line L592 (19.25, 29.5) -> (10.75, 29.5)
  line L593 (10.75, 29.5) -> (10.75, 28)
  line L594 (10.75, 30.5) -> (19.25, 30.5)
  line L595 (19.25, 30.5) -> (19.25, 32)
  line L596 (19.25, 32) -> (10.75, 32)
  line L597 (10.75, 32) -> (10.75, 30.5)
  line L598 (10.75, 43) -> (19.25, 43)
  line L599 (19.25, 43) -> (19.25, 44.5)
  line L600 (19.25, 44.5) -> (10.75, 44.5)
  line L601 (10.75, 44.5) -> (10.75, 43)
  line L602 (10.75, 45.5) -> (19.25, 45.5)
  line L603 (19.25, 45.5) -> (19.25, 47)
  line L604 (19.25, 47) -> (10.75, 47)
  line L605 (10.75, 47) -> (10.75, 45.5)
  line L606 (10.75, 58) -> (19.25, 58)
  line L607 (19.25, 58) -> (19.25, 59.5)
  line L608 (19.25, 59.5) -> (10.75, 59.5)
  line L609 (10.75, 59.5) -> (10.75, 58)
  line L610 (10.75, 60.5) -> (19.25, 60.5)
  line L611 (19.25, 60.5) -> (19.25, 62)
  line L612 (19.25, 62) -> (10.75, 62)
  line L613 (10.75, 62) -> (10.75, 60.5)
  line L614 (10.75, 73) -> (19.25, 73)
  line L615 (19.25, 73) -> (19.25, 74.5)
  line L616 (19.25, 74.5) -> (10.75, 74.5)
  line L617 (10.75, 74.5) -> (10.75, 73)
  line L618 (10.75, 75.5) -> (19.25, 75.5)
  line L619 (19.25, 75.5) -> (19.25, 77)
  line L620 (19.25, 77) -> (10.75, 77)
  line L621 (10.75, 77) -> (10.75, 75.5)
  line L622 (10.75, 88) -> (19.25, 88)
  line L623 (19.25, 88) -> (19.25, 89.5)
  line L624 (19.25, 89.5) -> (10.75, 89.5)
  line L625 (10.75, 89.5) -> (10.75, 88)
  line L626 (10.75, 90.5) -> (19.25, 90.5)
  line L627 (19.25, 90.5) -> (19.25, 92)
  line L628 (19.25, 92) -> (10.75, 92)
  line L629 (10.75, 92) -> (10.75, 90.5)
  line L630 (10.75, 103) -> (19.25, 103)
  line L631 (19.25, 103) -> (19.25, 104.5)
  line L632 (19.25, 104.5) -> (10.75, 104.5)
  line L633 (10.75, 104.5) -> (10.75, 103)
  line L634 (10.75, 105.5) -> (19.25, 105.5)
  line L635 (19.25, 105.5) -> (19.25, 107)
  line L636 (19.25, 107) -> (10.75, 107)
  line L637 (10.75, 107) -> (10.75, 105.5)
  line L638 (10.75, 118) -> (19.25, 118)
  line L639 (19.25, 118) -> (19.25, 119.5)
  line L640 (19.25, 119.5) -> (10.75, 119.5)
  line L641 (10.75, 119.5) -> (10.75, 118)
  line L642 (25.75, -119.5) -> (34.25, -119.5)
  line L643 (34.25, -119.5) -> (34.25, -118)
  line L644 (34.25, -118) -> (25.75, -118)
  line L645 (25.75, -118) -> (25.75, -119.5)
  line L646 (25.75, -107) -> (34.25, -107)
  line L647 (34.25, -107) -> (34.25, -105.5)
  line L648 (34.25, -105.5) -> (25.75, -105.5)
  line L649 (25.75, -105.5) -> (25.75, -107)
  line L650 (25.75, -104.5) -> (34.25, -104.5)
  line L651 (34.25, -104.5) -> (34.25, -103)
  line L652 (34.25, -103) -> (25.75, -103)
  line L653 (25.75, -103) -> (25.75, -104.5)
  line L654 (25.75, -92) -> (34.25, -92)
  line L655 (34.25, -92) -> (34.25, -90.5)
  line L656 (34.25, -90.5) -> (25.75, -90.5)
  line L657 (25.75, -90.5) -> (25.75, -92)
  line L658 (25.75, -89.5) -> (34.25, -89.5)
  line L659 (34.25, -89.5) -> (34.25, -88)
  line L660 (34.25, -88) -> (25.75, -88)
  line L661 (25.75, -88) -> (25.75, -89.5)
  line L662 (25.75, -77) -> (34.25, -77)
  line L663 (34.25, -77) -> (34.25, -75.5)
  line L664 (34.25, -75.5) -> (25.75, -75.5)
  line L665 (25.75, -75.5) -> (25.75, -77)
  line L666 (25.75, -74.5) -> (34.25, -74.5)
  line L667 (34.25, -74.5) -> (34.25, -73)
  line L668 (34.25, -73) -> (25.75, -73)
  line L669 (25.75, -73) -> (25.75, -74.5)
  line L670 (25.75, -62) -> (34.25, -62)
  line L671 (34.25, -62) -> (34.25, -60.5)
  line L672 (34.25, -60.5) -> (25.75, -60.5)
  line L673 (25.75, -60.5) -> (25.75, -62)
  line L674 (25.75, -59.5) -> (34.25, -59.5)
  line L675 (34.25, -59.5) -> (34.25, -58)
  line L676 (34.25, -58) -> (25.75, -58)
  line L677 (25.75, -58) -> (25.75, -59.5)
  line L678 (25.75, -47) -> (34.25, -47)
  line L679 (34.25, -47) -> (34.25, -45.5)
  line L680 (34.25, -45.5) -> (25.75, -45.5)
  line L681 (25.75, -45.5) -> (25.75, -47)
  line L682 (25.75, -44.5) -> (34.25, -44.5)
  line L683 (34.25, -44.5) -> (34.25, -43)
  line L684 (34.25, -43) -> (25.75, -43)
  line L685 (25.75, -43) -> (25.75, -44.5)
  line L686 (25.75, -32) -> (34.25, -32)
  line L687 (34.25, -32) -> (34.25, -30.5)
  line L688 (34.25, -30.5) -> (25.75, -30.5)
  line L689 (25.75, -30.5) -> (25.75, -32)
  line L690 (25.75, -29.5) -> (34.25, -29.5)
  line L691 (34.25, -29.5) -> (34.25, -28)
  line L692 (34.25, -28) -> (25.75, -28)
  line L693 (25.75, -28) -> (25.75, -29.5)
  line L694 (25.75, -17) -> (34.25, -17)
  line L695 (34.25, -17) -> (34.25, -15.5)
  line L696 (34.25, -15.5) -> (25.75, -15.5)
  line L697 (25.75, -15.5) -> (25.75, -17)
  line L698 (25.75, -14.5) -> (34.25, -14.5)
  line L699 (34.25, -14.5) -> (34.25, -13)
  line L700 (34.25, -13) -> (25.75, -13)
  line L701 (25.75, -13) -> (25.75, -14.5)
  line L702 (25.75, -2) -> (34.25, -2)
  line L703 (34.25, -2) -> (34.25, -0.5)
  line L704 (34.25, -0.5) -> (25.75, -0.5)
  line L705 (25.75, -0.5) -> (25.75, -2)
  line L706 (25.75, 0.5) -> (34.25, 0.5)
  line L707 (34.25, 0.5) -> (34.25, 2)
  line L708 (34.25, 2) -> (25.75, 2)
  line L709 (25.75, 2) -> (25.75, 0.5)
  line L710 (25.75, 13) -> (34.25, 13)
  line L711 (34.25, 13) -> (34.25, 14.5)
  line L712 (34.25, 14.5) -> (25.75, 14.5)
  line L713 (25.75, 14.5) -> (25.75, 13)
  line L714 (25.75, 15.5) -> (34.25, 15.5)
  line L715 (34.25, 15.5) -> (34.25, 17)
  line L716 (34.25, 17) -> (25.75, 17)
  line L717 (25.75, 17) -> (25.75, 15.5)
  line L718 (25.75, 28) -> (34.25, 28)
  line L719 (34.25, 28) -> (34.25, 29.5)
  line L720 (34.25, 29.5) -> (25.75, 29.5)
  line L721 (25.75, 29.5) -> (25.75, 28)
  line L722 (25.75, 30.5) -> (34.25, 30.5)
  line L723 (34.25, 30.5) -> (34.25, 32)
  line L724 (34.25, 32) -> (25.75, 32)
  line L725 (25.75, 32) -> (25.75, 30.5)
  line L726 (25.75, 43) -> (34.25, 43)
  line L727 (34.25, 43) -> (34.25, 44.5)
  line L728 (34.25, 44.5) -> (25.75, 44.5)
  line L729 (25.75, 44.5) -> (25.75, 43)
  line L730 (25.75, 45.5) -> (34.25, 45.5)
  line L731 (34.25, 45.5) -> (34.25, 47)
  line L732 (34.25, 47) -> (25.75, 47)
  line L733 (25.75, 47) -> (25.75, 45.5)
  line L734 (25.75, 58) -> (34.25, 58)
  line L735 (34.25, 58) -> (34.25, 59.5)
  line L736 (34.25, 59.5) -> (25.75, 59.5)
  line L737 (25.75, 59.5) -> (25.75, 58)
  line L738 (25.75, 60.5) -> (34.25, 60.5)
  line L739 (34.25, 60.5) -> (34.25, 62)
  line L740 (34.25, 62) -> (25.75, 62)
  line L741 (25.75, 62) -> (25.75, 60.5)
  line L742 (25.75, 73) -> (34.25, 73)
  line L743 (34.25, 73) -> (34.25, 74.5)
  line L744 (34.25, 74.5) -> (25.75, 74.5)
  line L745 (25.75, 74.5) -> (25.75, 73)
  line L746 (25.75, 75.5) -> (34.25, 75.5)
  line L747 (34.25, 75.5) -> (34.25, 77)
  line L748 (34.25, 77) -> (25.75, 77)
  line L749 (25.75, 77) -> (25.75, 75.5)
  line L750 (25.75, 88) -> (34.25, 88)
  line L751 (34.25, 88) -> (34.25, 89.5)
  line L752 (34.25, 89.5) -> (25.75, 89.5)
  line L753 (25.75, 89.5) -> (25.75, 88)
  line L754 (25.75, 90.5) -> (34.25, 90.5)
  line L755 (34.25, 90.5) -> (34.25, 92)
  line L756 (34.25, 92) -> (25.75, 92)
  line L757 (25.75, 92) -> (25.75, 90.5)
  line L758 (25.75, 103) -> (34.25, 103)
  line L759 (34.25, 103) -> (34.25, 104.5)
  line L760 (34.25, 104.5) -> (25.75, 104.5)
  line L761 (25.75, 104.5) -> (25.75, 103)
  line L762 (25.75, 105.5) -> (34.25, 105.5)
  line L763 (34.25, 105.5) -> (34.25, 107)
  line L764 (34.25, 107) -> (25.75, 107)
  line L765 (25.75, 107) -> (25.75, 105.5)
  line L766 (25.75, 118) -> (34.25, 118)
  line L767 (34.25, 118) -> (34.25, 119.5)
  line L768 (34.25, 119.5) -> (25.75, 119.5)
  line L769 (25.75, 119.5) -> (25.75, 118)
  line L770 (40.75, -119.5) -> (49.25, -119.5)
  line L771 (49.25, -119.5) -> (49.25, -118)
  line L772 (49.25, -118) -> (40.75, -118)
  line L773 (40.75, -118) -> (40.75, -119.5)
  line L774 (40.75, -107) -> (49.25, -107)
  line L775 (49.25, -107) -> (49.25, -105.5)
  line L776 (49.25, -105.5) -> (40.75, -105.5)
  line L777 (40.75, -105.5) -> (40.75, -107)
  line L778 (40.75, -104.5) -> (49.25, -104.5)
  line L779 (49.25, -104.5) -> (49.25, -103)
  line L780 (49.25, -103) -> (40.75, -103)
  line L781 (40.75, -103) -> (40.75, -104.5)
  line L782 (40.75, -92) -> (49.25, -92)
  line L783 (49.25, -92) -> (49.25, -90.5)
  line L784 (49.25, -90.5) -> (40.75, -90.5)
  line L785 (40.75, -90.5) -> (40.75, -92)
  line L786 (40.75, -89.5) -> (49.25, -89.5)
  line L787 (49.25, -89.5) -> (49.25, -88)
  line L788 (49.25, -88) -> (40.75, -88)
  line L789 (40.75, -88) -> (40.75, -89.5)
  line L790 (40.75, -77) -> (49.25, -77)
  line L791 (49.25, -77) -> (49.25, -75.5)
  line L792 (49.25, -75.5) -> (40.75, -75.5)
  line L793 (40.75, -75.5) -> (40.75, -77)
  line L794 (40.75, -74.5) -> (49.25, -74.5)
  line L795 (49.25, -74.5) -> (49.25, -73)
  line L796 (49.25, -73) -> (40.75, -73)
  line L797 (40.75, -73) -> (40.75, -74.5)
  line L798 (40.75, -62) -> (49.25, -62)
  line L799 (49.25, -62) -> (49.25, -60.5)
  line L800 (49.25, -60.5) -> (40.75, -60.5)
  line L801 (40.75, -60.5) -> (40.75, -62)
  line L802 (40.75, -59.5) -> (49.25, -59.5)
  line L803 (49.25, -59.5) -> (49.25, -58)
  line L804 (49.25, -58) -> (40.75, -58)
  line L805 (40.75, -58) -> (40.75, -59.5)
  line L806 (40.75, -47) -> (49.25, -47)
  line L807 (49.25, -47) -> (49.25, -45.5)
  line L808 (49.25, -45.5) -> (40.75, -45.5)
  line L809 (40.75, -45.5) -> (40.75, -47)
  line L810 (40.75, -44.5) -> (49.25, -44.5)
  line L811 (49.25, -44.5) -> (49.25, -43)
  line L812 (49.25, -43) -> (40.75, -43)
  line L813 (40.75, -43) -> (40.75, -44.5)
  line L814 (40.75, -32) -> (49.25, -32)
  line L815 (49.25, -32) -> (49.25, -30.5)
  line L816 (49.25, -30.5) -> (40.75, -30.5)
  line L817 (40.75, -30.5) -> (40.75, -32)
  line L818 (40.75, -29.5) -> (49.25, -29.5)
  line L819 (49.25, -29.5) -> (49.25, -28)
  line L820 (49.25, -28) -> (40.75, -28)
  line L821 (40.75, -28) -> (40.75, -29.5)
  line L822 (40.75, -17) -> (49.25, -17)
  line L823 (49.25, -17) -> (49.25, -15.5)
  line L824 (49.25, -15.5) -> (40.75, -15.5)
  line L825 (40.75, -15.5) -> (40.75, -17)
  line L826 (40.75, -14.5) -> (49.25, -14.5)
  line L827 (49.25, -14.5) -> (49.25, -13)
  line L828 (49.25, -13) -> (40.75, -13)
  line L829 (40.75, -13) -> (40.75, -14.5)
  line L830 (40.75, -2) -> (49.25, -2)
  line L831 (49.25, -2) -> (49.25, -0.5)
  line L832 (49.25, -0.5) -> (40.75, -0.5)
  line L833 (40.75, -0.5) -> (40.75, -2)
  line L834 (40.75, 0.5) -> (49.25, 0.5)
  line L835 (49.25, 0.5) -> (49.25, 2)
  line L836 (49.25, 2) -> (40.75, 2)
  line L837 (40.75, 2) -> (40.75, 0.5)
  line L838 (40.75, 13) -> (49.25, 13)
  line L839 (49.25, 13) -> (49.25, 14.5)
  line L840 (49.25, 14.5) -> (40.75, 14.5)
  line L841 (40.75, 14.5) -> (40.75, 13)
  line L842 (40.75, 15.5) -> (49.25, 15.5)
  line L843 (49.25, 15.5) -> (49.25, 17)
  line L844 (49.25, 17) -> (40.75, 17)
  line L845 (40.75, 17) -> (40.75, 15.5)
  line L846 (40.75, 28) -> (49.25, 28)
  line L847 (49.25, 28) -> (49.25, 29.5)
  line L848 (49.25, 29.5) -> (40.75, 29.5)
  line L849 (40.75, 29.5) -> (40.75, 28)
  line L850 (40.75, 30.5) -> (49.25, 30.5)
  line L851 (49.25, 30.5) -> (49.25, 32)
  line L852 (49.25, 32) -> (40.75, 32)
  line L853 (40.75, 32) -> (40.75, 30.5)
  line L854 (40.75, 43) -> (49.25, 43)
  line L855 (49.25, 43) -> (49.25, 44.5)
  line L856 (49.25, 44.5) -> (40.75, 44.5)
  line L857 (40.75, 44.5) -> (40.75, 43)
  line L858 (40.75, 45.5) -> (49.25, 45.5)
  line L859 (49.25, 45.5) -> (49.25, 47)
  line L860 (49.25, 47) -> (40.75, 47)
  line L861 (40.75, 47) -> (40.75, 45.5)
  line L862 (40.75, 58) -> (49.25, 58)
  line L863 (49.25, 58) -> (49.25, 59.5)
  line L864 (49.25, 59.5) -> (40.75, 59.5)
  line L865 (40.75, 59.5) -> (40.75, 58)
  line L866 (40.75, 60.5) -> (49.25, 60.5)
  line L867 (49.25, 60.5) -> (49.25, 62)
  line L868 (49.25, 62) -> (40.75, 62)
  line L869 (40.75, 62) -> (40.75, 60.5)
  line L870 (40.75, 73) -> (49.25, 73)
  line L871 (49.25, 73) -> (49.25, 74.5)
  line L872 (49.25, 74.5) -> (40.75, 74.5)
  line L873 (40.75, 74.5) -> (40.75, 73)
  line L874 (40.75, 75.5) -> (49.25, 75.5)
  line L875 (49.25, 75.5) -> (49.25, 77)
  line L876 (49.25, 77) -> (40.75, 77)
  line L877 (40.75, 77) -> (40.75, 75.5)
  line L878 (40.75, 88) -> (49.25, 88)
  line L879 (49.25, 88) -> (49.25, 89.5)
  line L880 (49.25, 89.5) -> (40.75, 89.5)
  line L881 (40.75, 89.5) -> (40.75, 88)
  line L882 (40.75, 90.5) -> (49.25, 90.5)
  line L883 (49.25, 90.5) -> (49.25, 92)
  line L884 (49.25, 92) -> (40.75, 92)
  line L885 (40.75, 92) -> (40.75, 90.5)
  line L886 (40.75, 103) -> (49.25, 103)
  line L887 (49.25, 103) -> (49.25, 104.5)
  line L888 (49.25, 104.5) -> (40.75, 104.5)
  line L889 (40.75, 104.5) -> (40.75, 103)
  line L890 (40.75, 105.5) -> (49.25, 105.5)
  line L891 (49.25, 105.5) -> (49.25, 107)
  line L892 (49.25, 107) -> (40.75, 107)
  line L893 (40.75, 107) -> (40.75, 105.5)
  line L894 (40.75, 118) -> (49.25, 118)
  line L895 (49.25, 118) -> (49.25, 119.5)
  line L896 (49.25, 119.5) -> (40.75, 119.5)
  line L897 (40.75, 119.5) -> (40.75, 118)
  line L898 (60.5, -128.5) -> (60.5, 128.5) projected
  line L899 (10.75, -69.5) -> (19.25, -69.5)
  line L900 (19.25, -69.5) -> (19.25, -68)
  line L901 (19.25, -68) -> (10.75, -68)
  line L902 (10.75, -68) -> (10.75, -69.5)
  line L903 (10.75, -67) -> (19.25, -67)
  line L904 (19.25, -67) -> (19.25, -65.5)
  line L905 (19.25, -65.5) -> (10.75, -65.5)
  line L906 (10.75, -65.5) -> (10.75, -67)
  line L907 (10.75, -24.5) -> (19.25, -24.5)
  line L908 (19.25, -24.5) -> (19.25, -23)
  line L909 (19.25, -23) -> (10.75, -23)
  line L910 (10.75, -23) -> (10.75, -24.5)
  line L911 (10.75, -22) -> (19.25, -22)
  line L912 (19.25, -22) -> (19.25, -20.5)
  line L913 (19.25, -20.5) -> (10.75, -20.5)
  line L914 (10.75, -20.5) -> (10.75, -22)
  line L915 (10.75, -9.5) -> (19.25, -9.5)
  line L916 (19.25, -9.5) -> (19.25, -8)
  line L917 (19.25, -8) -> (10.75, -8)
  line L918 (10.75, -8) -> (10.75, -9.5)
  line L919 (10.75, -7) -> (19.25, -7)
  line L920 (19.25, -7) -> (19.25, -5.5)
  line L921 (19.25, -5.5) -> (10.75, -5.5)
  line L922 (10.75, -5.5) -> (10.75, -7)
  line L923 (10.75, 35.5) -> (19.25, 35.5)
  line L924 (19.25, 35.5) -> (19.25, 37)
  line L925 (19.25, 37) -> (10.75, 37)
  line L926 (10.75, 37) -> (10.75, 35.5)
  line L927 (10.75, 38) -> (19.25, 38)
  line L928 (19.25, 38) -> (19.25, 39.5)
  line L929 (19.25, 39.5) -> (10.75, 39.5)
  line L930 (10.75, 39.5) -> (10.75, 38)
  line L931 (10.75, 80.5) -> (19.25, 80.5)
  line L932 (19.25, 80.5) -> (19.25, 82)
  line L933 (19.25, 82) -> (10.75, 82)
  line L934 (10.75, 82) -> (10.75, 80.5)
  line L935 (10.75, 83) -> (19.25, 83)
  line L936 (19.25, 83) -> (19.25, 84.5)
  line L937 (19.25, 84.5) -> (10.75, 84.5)
  line L938 (10.75, 84.5) -> (10.75, 83)
  line L939 (10.75, 95.5) -> (19.25, 95.5)
  line L940 (19.25, 95.5) -> (19.25, 97)
  line L941 (19.25, 97) -> (10.75, 97)
  line L942 (10.75, 97) -> (10.75, 95.5)
  line L943 (10.75, 98) -> (19.25, 98)
  line L944 (19.25, 98) -> (19.25, 99.5)
  line L945 (19.25, 99.5) -> (10.75, 99.5)
  line L946 (10.75, 99.5) -> (10.75, 98)
  point P0 (0, 0)
  dimension "d93" = 8.5
  dimension "d94" = 1.5
  dimension "d95" = 1.5
  dimension "d96" = 11
  dimension "d97" = 11.25
  dimension "d98" = 9
  dimension "d101" = 15
  dimension "d104" = 15
  dimension "d249" = 18.5
  dimension "d250" = 1.5
  dimension "d251" = 8.5
  dimension "d252" = 1.5
  dimension "d253" = 18.5
  dimension "d254" = 1.5
  dimension "d255" = 1.5
  dimension "d256" = 1.5
  dimension "d257" = 8.5
  dimension "d258" = 18.5
  dimension "d259" = 8.5
  dimension "d260" = 11
  dimension "d261" = 1
  dimension "d262" = 8.5
  dimension "d263" = 18.5
  dimension "d264" = 1.5
  dimension "d265" = 1.5
  dimension "d266" = 1.5
  dimension "d267" = 18.5
  dimension "d268" = 18.5
  dimension "d269" = 8.5
  dimension "d270" = 8.5
  dimension "d271" = 1.5
  dimension "d272" = 1.5
  dimension "d273" = 1.5
  dimension "d274" = 1.5
  dimension "d275" = 18.5
  dimension "d276" = 1
  dimension "d277" = 18.5
  dimension "d278" = 1
  dimension "d279" = 8.5
  dimension "d280" = 8.5
  dimension "d281" = 8.5
  dimension "d282" = 8.5
  constraints: 1888 end point, 238 point on line, 28 parallel, 15 horizontal, 14 perpendicular, 1 vertical, 1776 other
  measures "d93" distance of L5.end L6.end
  measures "d94" distance of L2.end L0.start
  measures "d95" distance of L6.end L4.start
  measures "d96" distance between parallel lines of L2 L4
  measures "d97" distance between parallel lines of L8 L3
  measures "d98" distance between parallel lines of L9 L0
  measures "d101" distance of L0.start L10.start
  measures "d104" distance of L0.start L130.start
  measures "d249" distance between parallel lines of L899 L532
  measures "d250" distance of L901.end L899.start
  measures "d251" distance between parallel lines of L539 L902
  measures "d252" distance of L905.end L903.start
  measures "d253" distance between parallel lines of L550 L905
  measures "d254" distance of L909.end L907.start
  measures "d255" distance of L913.end L911.start
  measures "d256" distance of L917.end L915.start
  measures "d257" distance between parallel lines of L545 L904
  measures "d258" distance between parallel lines of L556 L907
  measures "d259" distance between parallel lines of L563 L910
  measures "d260" distance between parallel lines of L915 L913
  measures "d261" distance between parallel lines of L909 L911
  measures "d262" distance between parallel lines of L565 L908
  measures "d263" distance between parallel lines of L582 L921
  measures "d264" distance of L919.end L920.end
  measures "d265" distance of L925.end L923.start
  measures "d266" distance of L929.end L927.start
  measures "d267" distance between parallel lines of L588 L923
  measures "d268" distance between parallel lines of L606 L929
  measures "d269" distance between parallel lines of L601 L928
  measures "d270" distance between parallel lines of L599 L930
  measures "d271" distance of L933.end L931.start
  measures "d272" distance of L937.end L935.start
  measures "d273" distance of L941.end L939.start
  measures "d274" distance of L945.end L943.start
  measures "d275" distance between parallel lines of L638 L945
  measures "d276" distance between parallel lines of L941 L943
  measures "d277" distance between parallel lines of L612 L931
  measures "d278" distance between parallel lines of L933 L935
  measures "d279" distance between parallel lines of L619 L934
  measures "d280" distance between parallel lines of L625 L932
  measures "d281" distance between parallel lines of L627 L942
  measures "d282" distance between parallel lines of L633 L944
extrude "Extrusion4" cut sketch "Sketch10" against normal through all contours L3 L2 L1 L0 | L7 L6 L5 L4 | L13 L12 L11 L10 | L17 L16 L15 L14 | L133 L132 L131 L130 | L137 L136 L135 L134 | L141 L140 L139 L138 | L145 L144 L143 L142 | L261 L260 L259 L258 | L265 L264 L263 L262 | L269 L268 L267 L266 | L273 L272 L271 L270 | L325 L324 L323 L322 | L329 L328 L327 L326 | L333 L332 L331 L330 | L337 L336 L335 L334 | L341 L340 L339 L338 | L345 L344 L343 L342 | L349 L348 L347 L346 | L353 L352 L351 L350 | L357 L356 L355 L354 | L361 L360 L359 L358 | L365 L364 L363 L362 | L369 L368 L367 L366 | L373 L372 L371 L370 | L377 L376 L375 L374 | L381 L380 L379 L378 | L385 L384 L383 L382 | L389 L388 L387 L386 | L393 L392 L391 L390 | L397 L396 L395 L394 | L401 L400 L399 L398 | L453 L452 L451 L450 | L457 L456 L455 L454 | L461 L460 L459 L458 | L465 L464 L463 L462 | L469 L468 L467 L466 | L473 L472 L471 L470 | L477 L476 L475 L474 | L481 L480 L479 L478 | L485 L484 L483 L482 | L489 L488 L487 L486 | L493 L492 L491 L490 | L497 L496 L495 L494 | L501 L500 L499 L498 | L505 L504 L503 L502 | L509 L508 L507 L506 | L513 L512 L511 L510 | L517 L516 L515 L514 | L521 L520 L519 L518 | L525 L524 L523 L522 | L529 L528 L527 L526 | L533 L532 L531 L530 | L553 L552 L551 L550 | L557 L556 L555 L554 | L585 L584 L583 L582 | L589 L588 L587 L586 | L609 L608 L607 L606 | L613 L612 L611 L610 | L641 L640 L639 L638 | L645 L644 L643 L642 | L649 L648 L647 L646 | L653 L652 L651 L650 | L657 L656 L655 L654 | L661 L660 L659 L658 | L665 L664 L663 L662 | L669 L668 L667 L666 | L673 L672 L671 L670 | L677 L676 L675 L674 | L681 L680 L679 L678 | L685 L684 L683 L682 | L689 L688 L687 L686 | L693 L692 L691 L690 | L697 L696 L695 L694 | L701 L700 L699 L698 | L705 L704 L703 L702 | L709 L708 L707 L706 | L713 L712 L711 L710 | L717 L716 L715 L714 | L721 L720 L719 L718 | L725 L724 L723 L722 | L729 L728 L727 L726 | L733 L732 L731 L730 | L737 L736 L735 L734 | L741 L740 L739 L738 | L745 L744 L743 L742 | L749 L748 L747 L746 | L753 L752 L751 L750 | L757 L756 L755 L754 | L761 L760 L759 L758 | L765 L764 L763 L762 | L769 L768 L767 L766 | L773 L772 L771 L770 | L777 L776 L775 L774 | L781 L780 L779 L778 | L785 L784 L783 L782 | L789 L788 L787 L786 | L793 L792 L791 L790 | L797 L796 L795 L794 | L801 L800 L799 L798 | L805 L804 L803 L802 | L809 L808 L807 L806 | L813 L812 L811 L810 | L817 L816 L815 L814 | L821 L820 L819 L818 | L825 L824 L823 L822 | L829 L828 L827 L826 | L833 L832 L831 L830 | L837 L836 L835 L834 | L841 L840 L839 L838 | L845 L844 L843 L842 | L849 L848 L847 L846 | L853 L852 L851 L850 | L857 L856 L855 L854 | L861 L860 L859 L858 | L865 L864 L863 L862 | L869 L868 L867 L866 | L873 L872 L871 L870 | L877 L876 L875 L874 | L881 L880 L879 L878 | L885 L884 L883 L882 | L889 L888 L887 L886 | L893 L892 L891 L890 | L897 L896 L895 L894 | L902 L901 L900 L899 | L906 L905 L904 L903 | L910 L909 L908 L907 | L914 L913 L912 L911 | L918 L917 L916 L915 | L922 L921 L920 L919 | L926 L925 L924 L923 | L930 L929 L928 L927 | L934 L933 L932 L931 | L938 L937 L936 L935 | L942 L941 L940 L939 | L946 L945 L944 L943